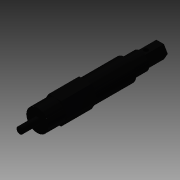
# Autodesk Inventor part: Carriage Shaft - Input
Saved by Autodesk Inventor 2013 (Build 170138000, 138)
## iProperties
Created: 2013-04-02
Part Number: Carriage Shaft - Input
Material: Generic
Document SubType Name: Modeling
Designer: mvarma
Density: 1 g/cm^3
Author: mvarma
Autodesk Inventor part; units mm, degrees
ref_plane "YZ Plane" through (0, 0, 0) normal (1, 0, 0) x (0, 1, 0)
ref_plane "XZ Plane" through (0, 0, 0) normal (0, 1, 0) x (-1, 0, 0)
ref_plane "XY Plane" through (0, 0, 0) normal (0, 0, 1) x (1, 0, 0)
sketch "Sketch1" plane through (0, 0, 0) normal (0, 0, 1) x (1, 0, 0)
  circle A0 centre (0, 0) radius 6.35
  dimension "d24" = 12.7
  constraints: 2 coincident, 1 centre point
  measures "d24" diameter of A0
extrude "Extrusion1" add sketch "Sketch1" along normal blind 11.1125
sketch "Sketch7" plane through (0, 0, 0) normal (0, 0, -1) x (-1, 0, 0)
  circle A0 centre (0, 0) radius 6.35 projected
  line L0 (-5.4993, 0) -> (-2.7496, 4.7625)
  line L1 (-2.7496, 4.7625) -> (2.7496, 4.7625)
  line L2 (2.7496, 4.7625) -> (5.4993, 0)
  line L3 (5.4993, 0) -> (2.7496, -4.7625)
  line L4 (2.7496, -4.7625) -> (-2.7496, -4.7625)
  line L5 (-2.7496, -4.7625) -> (-5.4993, 0)
  dimension "d26" = 9.525
  constraints: 12 end point, 1 coincident, 1 horizontal, 13 other
  measures "d26" distance between parallel lines of L4 L1
extrude "Extrusion7" add sketch "Sketch7" along normal blind 14.2454 contours L0 L1 L2 L3 L4 L5
sketch "Sketch4" plane through (0, 0, 11.1125) normal (0, 0, 1) x (1, 0, 0)
  circle A0 centre (0, 0) radius 7.9375
  dimension "d10" = 15.875
  constraints: 1 centre point, 1 coincident
  measures "d10" diameter of A0
extrude "Extrusion4" add sketch "Sketch4" along normal blind 28.9719
sketch "Sketch9" plane through (0, 0, 40.0844) normal (0, 0, 1) x (1, 0, 0)
  circle A0 centre (0, 0) radius 7.9375 projected
  line L0 (-9.1654, 0) -> (-4.5827, 7.9375)
  line L1 (-4.5827, 7.9375) -> (4.5827, 7.9375)
  line L2 (4.5827, 7.9375) -> (9.1654, 0)
  line L3 (9.1654, 0) -> (4.5827, -7.9375)
  line L4 (4.5827, -7.9375) -> (-4.5827, -7.9375)
  line L5 (-4.5827, -7.9375) -> (-9.1654, 0)
  dimension "d34" = 15.875
  constraints: 12 end point, 1 coincident, 1 horizontal, 13 other
  measures "d34" distance between parallel lines of L4 L1
extrude "Extrusion9" add sketch "Sketch9" along normal blind 22.225
sketch "Sketch8" plane through (-2.7496, 4.7625, 0) normal (0, 1, 0) x (1, 0, 0)
  line L0 (5.4993, 0) -> (0, 0) projected
  line L1 (0, 14.2454) -> (5.4993, 14.2454) projected
  line L2 (2.7496, 14.2454) -> (2.7496, 0) construction
  circle A0 centre (2.7496, 3.9688) radius 1.5875
  dimension "d29" = 3.175
  dimension "d31" = 3.9688
  constraints: 2 end point, 1 centre point, 1 midpoint, 1 perpendicular, 1 point on line
  measures "d29" diameter of A0
  measures "d31" distance from line of L0 A0.centre
extrude "Extrusion8" cut sketch "Sketch8" against normal through all
sketch "Sketch10" plane through (0, 0, 62.3094) normal (0, 0, 1) x (1, 0, 0)
  line L0 (-4.5827, 7.9375) -> (-9.1654, 0) projected
  circle A0 centre (0, 0) radius 7.9375
  constraints: 1 centre point, 1 coincident, 1 tangent
extrude "Extrusion10" add sketch "Sketch10" along normal blind 12.7
sketch "Sketch11" plane through (0, 0, 75.0094) normal (0, 0, 1) x (1, 0, 0)
  circle A0 centre (0, 0) radius 7.9375 projected
  circle A1 centre (0, 0) radius 2.3813
  dimension "d39" = 4.7625
  constraints: 1 centre point, 1 coincident
  measures "d39" diameter of A1
extrude "Extrusion11" add sketch "Sketch11" along normal blind 12.7 contours A1
body "Solid1"
